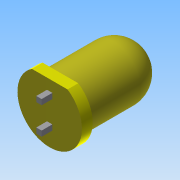
# Autodesk Inventor part: LED
Saved by Autodesk Inventor 2016 (Build 200138000, 138)
## iProperties
Created: 2015-06-12
Part Number: LED
Material: Generic
Document SubType Name: Modeling
Designer: Openlab
Density: 1 g/cm^3
Appearance: Default
Author: Openlab
Autodesk Inventor part; units mm, degrees
ref_plane "YZ Plane" through (0, 0, 0) normal (1, 0, 0) x (0, 1, 0)
ref_plane "XZ Plane" through (0, 0, 0) normal (0, 1, 0) x (-1, 0, 0)
ref_plane "XY Plane" through (0, 0, 0) normal (0, 0, 1) x (1, 0, 0)
sketch "Sketch1" plane through (0, 0, 0) normal (0, 1, 0) x (-1, 0, 0)
  arc A0 (-1.6583, 2.5) -> (1.6583, 2.5) centre (0, 0) ccw
  circle A1 centre (0, 0) radius 2.5
  line L0 (-1.6583, 2.5) -> (1.6583, 2.5)
  dimension "d0" = 6
  dimension "d1" = 5
  constraints: 2 centre point, 2 end point, 2 point on circle, 1 coincident, 1 horizontal, 1 tangent
  measures "d0" diameter of A0
  measures "d1" diameter of A1
extrude "Extrusion3" add sketch "Sketch1" along normal blind 1 contours A1 | L0 A0
sketch "Sketch2" plane through (0, 1, 0) normal (0, 1, 0) x (1, 0, 0)
  circle A0 centre (0, 0) radius 2.5 projected
  point P0 (0, -2.5)
  constraints: 1 vertical alignment
extrude "Extrusion5" add sketch "Sketch2" along normal blind 7.5
fillet "Fillet2" radius 2.5 1 edges at (-2.5, 8.5, 0)
sketch "Sketch3" plane through (0, 0, 0) normal (0, -1, 0) x (1, 0, 0)
  line L0 (-0.25, 1.52) -> (0.25, 1.52)
  line L1 (0.25, 1.52) -> (0.25, 1.02)
  line L2 (0.25, 1.02) -> (-0.25, 1.02)
  line L3 (-0.25, 1.02) -> (-0.25, 1.52)
  line L4 (-0.25, -1.02) -> (0.25, -1.02)
  line L5 (0.25, -1.02) -> (0.25, -1.52)
  line L6 (0.25, -1.52) -> (-0.25, -1.52)
  line L7 (-0.25, -1.52) -> (-0.25, -1.02)
  line L8 (-0.3964, 1.27) -> (0.6648, 1.27) construction
  line L9 (-0.5129, -1.27) -> (0.7016, -1.27) construction
  line L10 (-1.0602, 0) -> (0.7998, 0) construction
  point P0 (0, 0)
  point P1 (0.25, -1.27)
  point P2 (0.25, 1.27)
  point P3 (0, 1.02)
  dimension "d18" = 0.5
  dimension "d19" = 2.54
  constraints: 22 end point, 5 horizontal, 5 perpendicular, 4 parallel, 4 point on line, 3 midpoint, 1 vertical alignment, 1 other
  measures "d18" distance of L5.end L6.end
  measures "d19" distance between parallel lines of L9 L8
extrude "Extrusion6" add sketch "Sketch3" along normal blind 1
body "Solid1"
